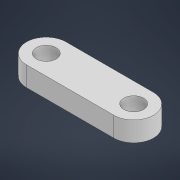
# Autodesk Inventor part: holder3_l3
Saved by Autodesk Inventor 2021 (Build 250183000, 183)
## iProperties
Created: 2021-06-13
Part Number: holder3_l3
Material: Generic
Document SubType Name: Modeling
Designer: Watchdog
Density: 1 g/cm^3
Appearance: Default
Author: Watchdog
Autodesk Inventor part; units mm, degrees
ref_plane "YZ Plane" through (0, 0, 0) normal (1, 0, 0) x (0, 1, 0)
ref_plane "XZ Plane" through (0, 0, 0) normal (0, 1, 0) x (-1, 0, 0)
ref_plane "XY Plane" through (0, 0, 0) normal (0, 0, 1) x (1, 0, 0)
sketch "Sketch1" plane through (0, 0, 0) normal (0, 1, 0) x (-1, 0, 0)
  line L0 (-7.8131, -4) -> (-25.4991, -4)
  line L1 (-25.4991, 4) -> (-7.8131, 4)
  arc A0 (-7.8131, -4) -> (-7.8131, 4) centre (-7.8131, 0) ccw
  arc A1 (-25.4991, 4) -> (-25.4991, -4) centre (-25.4991, 0) ccw
  point P0 (0, 0)
  dimension "d0" = 8
  dimension "d1" = 4
  dimension "d2" = 17.686
  constraints: 4 end point, 4 point on circle, 4 tangent, 2 centre point, 1 horizontal, 1 parallel
  measures "d0" distance between parallel lines of L1 L0
  measures "d1" distance from line of point (0, 0) L0
  measures "d2" distance of L0.end L0.start
extrude "Extrusion1" add sketch "Sketch1" along normal blind 4
sketch "Sketch2" plane through (0, 4, 0) normal (0, 1, 0) x (1, 0, 0)
  arc A0 (7.8131, 4) -> (7.8131, -4) centre (7.8131, 0) ccw projected
  arc A1 (25.4991, -4) -> (25.4991, 4) centre (25.4991, 0) ccw projected
  point P0 (0, 0)
  dimension "d5" = 0
  dimension "d6" = 0
  dimension "d7" = 0
  dimension "d8" = 0
  measures "d5" distance of A0.centre point (7.813, 0)
  measures "d6" distance of A0.centre point (7.813, 0)
  measures "d7" distance of A1.centre point (25.499, 0)
  measures "d8" distance of A1.centre point (25.499, 0)
hole "Hole1" at (7.8131, 4, 0) at (25.4991, 4, 0) direction (0, -1, 0) diameter 4 end through all
equation "\"d1\" = 0.5 * d0"
body "Solid1"
